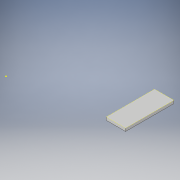
# Autodesk Inventor part: Tape Measure Holder attachment
Saved by Autodesk Inventor 2019 (Build 230136000, 136)
## iProperties
Created: 2018-11-14
Part Number: Tape Measure Holder attachment
Material: Generic
Document SubType Name: Modeling
Designer: Ashley
Density: 1 g/cm^3
Appearance: Default
Author: Ashley
Autodesk Inventor part; units mm, degrees
ref_plane "YZ Plane" through (0, 0, 0) normal (1, 0, 0) x (0, 1, 0)
ref_plane "XZ Plane" through (0, 0, 0) normal (0, 1, 0) x (-1, 0, 0)
ref_plane "XY Plane" through (0, 0, 0) normal (0, 0, 1) x (1, 0, 0)
sketch "Sketch1" plane through (0, 0, 0) normal (0, 1, 0) x (-1, 0, 0)
  line L0 (-108.2064, -15.48) -> (-88.2064, -15.48)
  line L1 (-88.2064, -15.48) -> (-88.2064, -65.48)
  line L2 (-88.2064, -65.48) -> (-108.2064, -65.48)
  line L3 (-108.2064, -65.48) -> (-108.2064, -15.48)
  point P0 (0, 0)
  dimension "d0" = 20
  dimension "d1" = 50
  constraints: 8 end point, 2 parallel, 1 horizontal, 1 perpendicular
  measures "d0" distance of L0.start L1.start
  measures "d1" distance of L1.start L1.end
extrude "Extrusion1" add sketch "Sketch1" along normal blind 3
sketch "Sketch2" plane through (0, 3, 0) normal (0, 1, 0) x (1, 0, 0)
  line L0 (88.2064, 15.48) -> (108.2064, 15.48) construction
  line L1 (108.2064, 15.48) -> (108.2064, 65.48) construction
  line L2 (108.2064, 65.48) -> (88.2064, 65.48) construction
  line L3 (88.2064, 65.48) -> (88.2064, 15.48) construction
  point P0 (0, 0)
body "Solid1"
